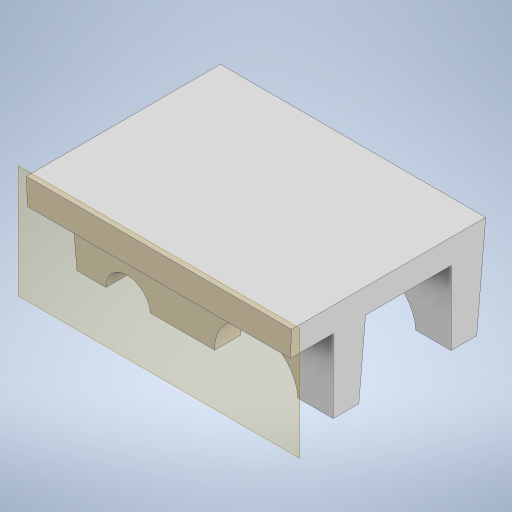
# Autodesk Inventor part: E.Engine Block Bottom Cast Image Right
Saved by Autodesk Inventor 2023 (Build 270158000, 158)
## iProperties
Created: 2023-01-04
Part Number: E.Engine Block Bottom Cast Image Right
Material: Generic
Document SubType Name: Modeling
Designer: tgr41
Density: 1 g/cm^3
Appearance: Default
Mass: 1928.08 g
Surface Area: 1645.68 cm^2
Volume: 1928.08 cm^3
Author: tgr41
Autodesk Inventor part; units mm, degrees
ref_plane "YZ Plane" through (0, 0, 0) normal (1, 0, 0) x (0, 1, 0)
ref_plane "XZ Plane" through (0, 0, 0) normal (0, 1, 0) x (-1, 0, 0)
ref_plane "XY Plane" through (0, 0, 0) normal (0, 0, 1) x (1, 0, 0)
sketch "Sketch1" plane through (0, 0, 0) normal (0, 0, 1) x (1, 0, 0)
  line L0 (127, 0) -> (127, 50.8)
  line L1 (127, 50.8) -> (0, 50.8)
  line L2 (0, 50.8) -> (0, 0)
  arc A0 (109.5375, 0) -> (68.2625, 0) centre (88.9, 0) ccw
  arc A1 (36.3964, 0) -> (14.4, 0) centre (25.3982, 0) ccw
  line L3 (14.4, 0) -> (0, 0)
  line L4 (127, 0) -> (109.5375, 0)
  line L5 (68.2625, 0) -> (36.3964, 0)
  dimension "d0" = 127
  dimension "d2" = 41.275
  dimension "d25" = 38.1
  dimension "d26" = 21.9964
  dimension "d31" = 31.8661
  dimension "d32" = 14.4
  dimension "d33" = 50.8
  constraints: 12 end point, 4 point on circle, 3 parallel, 2 centre point, 2 collinear, 1 perpendicular
  measures "d0" distance of L1.end L0.end
  measures "d2" diameter of A0
  measures "d25" distance from line of L0 A0.centre
  measures "d26" diameter of A1
  measures "d31" distance of L5.start L5.end
  measures "d32" distance of L3.start L2.end
  measures "d33" distance of L1.end L2.end
extrude "Extrusion1" add sketch "Sketch1" along normal blind 187.96
sketch "Sketch3" plane through (127, 0, 0) normal (1, 0, 0) x (0, 0, -1)
  line L0 (0, 50.8) -> (-187.96, 50.8) projected
  line L1 (0, 0) -> (-187.96, 0) projected
  line L2 (-35.56, 38.1) -> (-35.56, 0)
  line L3 (0, 0) -> (-187.96, 0) projected
  line L4 (-93.98, 0) -> (-93.98, 38.1)
  line L5 (-152.4, 38.1) -> (-152.4, 0)
  line L6 (0, 0) -> (0, 50.8) projected
  line L7 (-187.96, 0) -> (-175.26, 0)
  line L8 (-175.26, 0) -> (-175.26, 38.1)
  line L9 (-175.26, 50.8) -> (-187.96, 50.8)
  line L10 (-187.96, 50.8) -> (-187.96, 0)
  line L11 (-116.84, 0) -> (-129.54, 0)
  line L12 (-129.54, 0) -> (-129.54, 38.1)
  line L13 (-129.54, 50.8) -> (-116.84, 50.8)
  line L14 (-116.84, 38.1) -> (-116.84, 0)
  line L15 (-35.56, 38.1) -> (-35.56, 0)
  line L16 (0, 0) -> (-12.7, 0)
  line L17 (-12.7, 0) -> (-12.7, 38.1)
  line L18 (-12.7, 50.8) -> (0, 50.8)
  line L19 (0, 50.8) -> (0, 0)
  line L20 (-71.12, 0) -> (-58.42, 0)
  line L21 (-58.42, 0) -> (-58.42, 38.1)
  line L22 (-58.42, 50.8) -> (-71.12, 50.8)
  line L23 (-71.12, 38.1) -> (-71.12, 0)
  line L24 (-187.96, 50.8) -> (-187.96, 0) projected
  line L25 (-187.96, 50.8) -> (0, 50.8)
  line L26 (-58.42, 38.1) -> (-12.7, 38.1)
  line L27 (-175.26, 38.1) -> (-129.54, 38.1)
  line L28 (-116.84, 38.1) -> (-71.12, 38.1)
  dimension "d15" = 35.56
  dimension "d16" = 93.98
  dimension "d17" = 152.4
  dimension "d18" = 12.7
  dimension "d34" = 38.1
  constraints: 48 end point, 14 symmetric about line, 7 parallel, 7 perpendicular, 4 midpoint, 3 point on line, 2 horizontal
  measures "d15" distance between parallel lines of L6 L2
  measures "d16" distance between parallel lines of L6 L4
  measures "d17" distance between parallel lines of L6 L5
  measures "d18" distance of L9.end L9.start
  measures "d34" distance of L7.end L8.end
extrude "Extrusion2" cut sketch "Sketch3" against normal blind 187.96 contours L1 L2 L26 L17 | L1 L21 L26 L2 | L1 L4 L28 L23 | L1 L14 L28 L4 | L1 L5 L27 L12 | L8 L27 L5 L1
ref_plane "Work Plane1" through (0, 0, 93.98) normal (0, 0, 1) x (1, 0, 0)
sketch "Sketch5" plane through (0, 0, 93.98) normal (0, 0, 1) x (1, 0, 0)
  line L0 (139.1351, 65.2471) -> (-26.9806, 65.2471)
  line L1 (-26.9806, 65.2471) -> (-26.9806, -18.3397)
  line L2 (-26.9806, -18.3397) -> (139.1351, -18.3397)
  line L3 (139.1351, -18.3397) -> (139.1351, 65.2471)
  point P0 (0, 0)
  constraints: 8 end point, 2 parallel, 1 horizontal, 1 perpendicular
draft "FaceDraft1" angle 2.5 pull direction (0, -1, 0) fixed plane through (57.6405, 0, 62.6533) normal (0, -1, 0) faces at (71.1375, 32.229, 71.12) (71.1375, 32.229, 129.54) (69.5273, 40.2988, 187.96) (71.1375, 32.229, 12.7) (71.1375, 32.229, 175.26) (71.1375, 32.229, 116.84) (71.1375, 32.229, 58.42) (69.5273, 40.2988, 0) (0, 46.5667, 86.36) (127, 46.5667, 86.36)
extrude "Extrusion5" cut sketch "Sketch5" along normal blind 228.6
body "Solid1"
